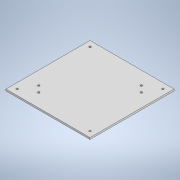
# Autodesk Inventor part: Base Plate
Saved by Autodesk Inventor 2022 (Build 260153000, 153)
## iProperties
Created: 2023-02-05
Part Number: Base Plate
Material: Generic
Document SubType Name: Modeling
Designer: Rishi  Agrawal
Density: 1 g/cm^3
Appearance: Default
Author: Rishi  Agrawal
Autodesk Inventor part; units mm, degrees
ref_plane "YZ Plane" through (0, 0, 0) normal (1, 0, 0) x (0, 1, 0)
ref_plane "XZ Plane" through (0, 0, 0) normal (0, 1, 0) x (-1, 0, 0)
ref_plane "XY Plane" through (0, 0, 0) normal (0, 0, 1) x (1, 0, 0)
sketch "Sketch1" plane through (0, 0, 0) normal (0, 1, 0) x (-1, 0, 0)
  line L0 (-150, 150) -> (150, 150)
  line L1 (150, 150) -> (150, -150)
  line L2 (150, -150) -> (-150, -150)
  line L3 (-150, -150) -> (-150, 150)
  line L4 (-150, 150) -> (150, -150) construction
  line L5 (150, 150) -> (-150, -150) construction
  point P0 (0, 0)
  dimension "d0" = 300
  dimension "d1" = 300
  constraints: 12 end point, 2 midpoint, 2 parallel, 1 horizontal, 1 perpendicular
  measures "d0" distance of L1.end L2.end
  measures "d1" distance of L0.end L1.end
extrude "Extrusion1" add sketch "Sketch1" along normal blind 6
sketch "Sketch2" plane through (0, 6, 0) normal (0, 1, 0) x (1, 0, 0)
  line L0 (-150, -150) -> (150, -150) projected
  line L1 (150, 150) -> (-150, 150) projected
  line L2 (-150, 150) -> (-150, -150) projected
  line L3 (-150, 150) -> (150, -150) construction
  line L4 (0, 0) -> (-91.5703, -91.5703) construction
  line L5 (0, 0) -> (129.5, 0) construction
  line L6 (-91.5703, -91.5703) -> (-102.1769, -80.9637) construction
  circle A0 centre (-102.1769, -80.9637) radius 3.35
  line L7 (-91.5703, -91.5703) -> (-80.9637, -102.1769) construction
  circle A1 centre (-80.9637, -102.1769) radius 3.35
  circle A2 centre (80.9637, 102.1769) radius 3.35
  circle A3 centre (102.1769, 80.9637) radius 3.35
  dimension "d4" = 129.5
  dimension "d5" = 135
  dimension "d6" = 15
  dimension "d7" = 6.7
  constraints: 10 end point, 4 centre point, 4 symmetric about line, 2 coincident, 1 equal length, 1 horizontal, 3 other
  measures "d4" distance of L4.start L4.end
  measures "d5" angle of L4 L5
  measures "d6" distance of L4.end L6.end
  measures "d7" diameter of A0
extrude "Extrusion2" cut sketch "Sketch2" against normal through all
sketch "Sketch3" plane through (0, 6, 0) normal (0, 1, 0) x (1, 0, 0)
  line L0 (-150, 150) -> (-150, -150) projected
  point P0 (0, 0)
  point P1 (-130, -130)
  point P2 (-130, 130)
  point P3 (130, 130)
  point P4 (130, -130)
  dimension "d17" = 20
  measures "d17" distance from line of L0 point (-130, 130)
hole "Hole1" at (-130, 6, 130) at (-130, 6, -130) at (130, 6, -130) at (130, 6, 130) direction (0, -1, 0) diameter 6.5 end through all
body "Solid1"
